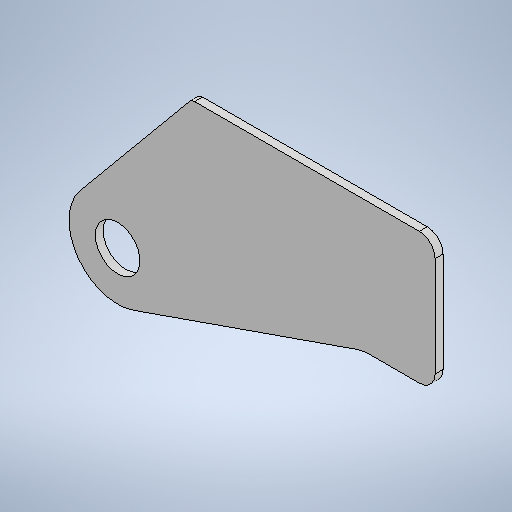
# Autodesk Inventor part: NDM-VOS Пятка под стойки
Saved by Autodesk Inventor 2025 (Build 290162010, 162A)
## iProperties
Created: 2024-07-01
Part Number: NDM-VOS Пятка под стойки
Material: Stainless Steel
Document SubType Name: Sheet Metal
Designer: pokla
Stock Number: МОО 901 базовая пластина
Mass: 271.203 g
Surface Area: 241.038 cm^2
Volume: 33.9004 cm^3
Density: 8 g/cm^3
Flat Pattern Width: 11.9182 cm
Flat Pattern Length: 12.6176 cm
Flat Pattern Area: 150.379 cm^2
Sheet Metal Rule: AISI304 4mm Die 32
Sheet Metal Width: 119,182 mm
Sheet Metal Length: 126,176 mm
Sheet Metal Area: 15037,931 mm^2
Appearance: Default
Author: pokla
Autodesk Inventor part; units mm, degrees
ref_plane "YZ Plane" through (0, 0, 0) normal (1, 0, 0) x (0, 1, 0)
ref_plane "XZ Plane" through (0, 0, 0) normal (0, 1, 0) x (-1, 0, 0)
ref_plane "XY Plane" through (0, 0, 0) normal (0, 0, 1) x (1, 0, 0)
sketch "Sketch1" plane through (0, 0, 0) normal (0, 1, 0) x (-1, 0, 0)
  line L0 (40, 20) -> (-40, 20) construction
  line L1 (-40, 20) -> (-40, -20) construction
  line L2 (-40, -20) -> (40, -20) construction
  line L3 (40, -20) -> (40, 20) construction
  line L4 (-40, 20) -> (40, -20) construction
  line L5 (0, 20) -> (0, -20) construction
  line L6 (-45, -25) -> (-45, 0)
  line L7 (-20, -25) -> (-45, -25)
  arc A0 (69.6915, -55.359) -> (90.0175, -26.0792) centre (75.7771, -37.8885) ccw
  circle A1 centre (75.7771, -37.8885) radius 8.5
  line L8 (69.6915, -55.359) -> (-15.0657, -25.8348)
  arc A2 (-15.0657, -25.8348) -> (-20, -25) centre (-20, -40) ccw
  arc A3 (90.0175, -26.0792) -> (69.6915, -55.359) centre (75.7771, -37.8885) ccw construction
  line L9 (-45, 0) -> (-45, 25)
  line L10 (-45, 25) -> (46.484, 25)
  line L11 (40, 0) -> (45, 0) construction
  line L12 (0, 20) -> (0, 25) construction
  line L13 (-40, 0) -> (-45, 0) construction
  line L14 (47.6585, 25) -> (48.4083, 24.0959) construction
  arc A4 (48.4083, 24.0959) -> (46.484, 25) centre (46.484, 22.5) ccw
  arc A5 (46.484, 25) -> (48.4083, 24.0959) centre (46.484, 22.5) ccw construction
  line L15 (48.4083, 24.0959) -> (90.0175, -26.0792)
  line L16 (46.484, 25) -> (47.6585, 25) construction
  point P0 (0, 0)
  point P1 (0, 0)
  point P2 (0, 0)
  dimension "d2" = 80
  dimension "d3" = 40
  dimension "d29" = 5
  dimension "d30" = 17
  dimension "d31" = 10
  dimension "d32" = 40
  dimension "d34" = 5
  dimension "d35" = 15
  dimension "d36" = 25
  dimension "d38" = 5
  dimension "d41" = 66.3579
  measures "d2" distance of L2.end L1.end
  measures "d3" distance of L1.end L0.end
  measures "d29" distance between parallel lines of L6 L1
  measures "d30" diameter of A1
  measures "d31" radial gap between concentric circles of A0 A1
  measures "d32" distance of L2.end A1.centre
  measures "d34" distance between parallel lines of L2 L7
  measures "d35" radius of A2
  measures "d36" distance of L7.start L6.start
  measures "d38" diameter of A4
  measures "d41" distance of L15.end L14.start
extrude "Plate1" add sketch "Sketch1" along normal blind 3
fillet "Corner Round3" radius 6 2 edges at (45, 1.5, 25) (45, 1.5, -25)
equation "\"d34\" = d29"
equation "\"d6\" = Thickness"
equation "\"Thickness\" = 3"
body "Solid1"
